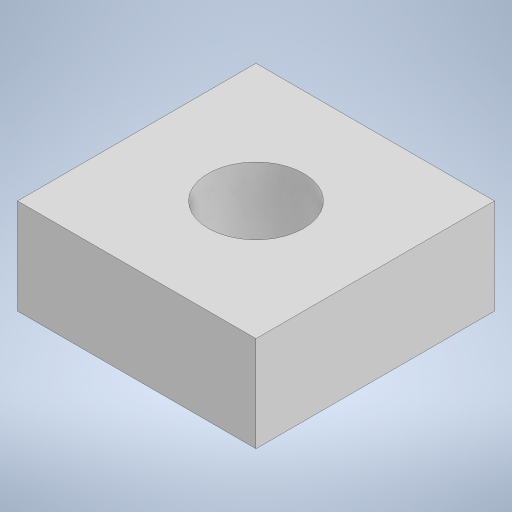
# Autodesk Inventor part: Holder
Saved by Autodesk Inventor 2024 (Build 280153000, 153)
## iProperties
Created: 2023-12-17
Part Number: Holder
Material: Generic
Document SubType Name: Modeling
Designer: pratikhya
Density: 1 g/cm^3
Appearance: Default
Author: pratikhya
Autodesk Inventor part; units mm, degrees
ref_plane "YZ Plane" through (0, 0, 0) normal (1, 0, 0) x (0, 1, 0)
ref_plane "XZ Plane" through (0, 0, 0) normal (0, 1, 0) x (-1, 0, 0)
ref_plane "XY Plane" through (0, 0, 0) normal (0, 0, 1) x (1, 0, 0)
sketch "Sketch6" plane through (0, 0, 0) normal (0, 1, 0) x (-1, 0, 0)
  line L0 (-3.75, -3.75) -> (3.75, -3.75)
  line L1 (3.75, -3.75) -> (3.75, 3.75)
  line L2 (3.75, 3.75) -> (-3.75, 3.75)
  line L3 (-3.75, 3.75) -> (-3.75, -3.75)
  line L4 (-3.75, -3.75) -> (3.75, 3.75) construction
  line L5 (3.75, -3.75) -> (-3.75, 3.75) construction
  point P0 (0, 0)
  dimension "d4" = 7.5
  dimension "d5" = 7.5
  constraints: 12 end point, 2 midpoint, 2 parallel, 1 horizontal, 1 perpendicular
  measures "d4" distance of L2.end L1.end
  measures "d5" distance of L1.end L0.end
extrude "Extrusion2" add sketch "Sketch6" along normal blind 10
sketch "Sketch7" plane through (3.75, 0, 3.75) normal (1, 0, 0) x (0, 0, -1)
  line L0 (7.5, 0) -> (0, 0) projected
  line L1 (0, 0) -> (7.5, 0)
  line L2 (0, 0) -> (0, 7)
  line L3 (0, 7) -> (7.5, 7)
  line L4 (7.5, 7) -> (7.5, 0)
  line L5 (7.5, 0) -> (0, 0)
  line L6 (0, 0) -> (0, 10) projected
  line L7 (7.5, 0) -> (7.5, 10) projected
  point P0 (3.75, 0)
  dimension "d9" = 7
  dimension "d19" = 0
  dimension "d20" = 0
  constraints: 10 end point, 2 point on line, 1 perpendicular, 1 vertical
  measures "d9" distance of L1.start L2.end
  measures "d19" distance between parallel lines of L6 L2
  measures "d20" distance between parallel lines of L7 L4
extrude "Extrusion3" cut sketch "Sketch7" against normal blind 9.05
sketch "Sketch8" plane through (0, 10, 0) normal (0, 1, 0) x (1, 0, 0)
  circle A0 centre (0, 0) radius 1.5
  dimension "d13" = 3
  constraints: 1 centre point, 1 coincident
  measures "d13" diameter of A0
extrude "Extrusion4" cut sketch "Sketch8" against normal blind 5.2375
body "Solid2"
